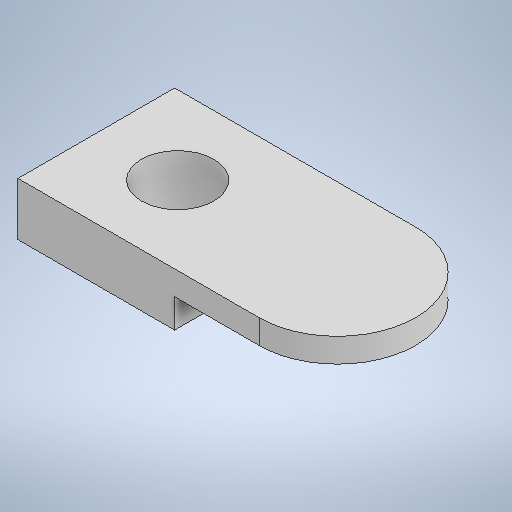
# Autodesk Inventor part: pinub
Saved by Autodesk Inventor 2025 (Build 290162000, 162)
## iProperties
Created: 2025-05-31
Part Number: pinub
Material: Generic
Document SubType Name: Modeling
Designer: ethan
Density: 1 g/cm^3
Appearance: Default
Author: ethan
Autodesk Inventor part; units mm, degrees
ref_plane "YZ Plane" through (0, 0, 0) normal (1, 0, 0) x (0, 1, 0)
ref_plane "XZ Plane" through (0, 0, 0) normal (0, 1, 0) x (-1, 0, 0)
ref_plane "XY Plane" through (0, 0, 0) normal (0, 0, 1) x (1, 0, 0)
sketch "Sketch1" plane through (0, 0, 0) normal (0, 1, 0) x (-1, 0, 0)
  line L0 (0, 0) -> (10, 0)
  line L1 (10, 0) -> (10, -6.5)
  line L2 (10, -6.5) -> (0, -6.5)
  line L3 (0, -6.5) -> (0, 0)
  arc A0 (0, 0) -> (0, -6.5) centre (0, -3.25) ccw
  dimension "d1" = 6.5
  dimension "d2" = 10
  constraints: 8 end point, 2 parallel, 2 point on circle, 2 tangent, 1 centre point, 1 horizontal, 1 perpendicular
  measures "d1" distance of L0.end L1.end
  measures "d2" distance of L1.end L2.end
extrude "Extrusion1" add sketch "Sketch1" along normal blind 1
sketch "Sketch2" plane through (0, 0, 0) normal (0, -1, 0) x (1, 0, 0)
  line L0 (-10, -6.5) -> (-10, 0) construction
  line L1 (0, -6.5) -> (-10, -6.5) construction
  arc A0 (0, -6.5) -> (0, 0) centre (0, -3.25) ccw construction
  line L2 (-10, 0) -> (0, 0) construction
  line L3 (-10, 0) -> (-3.5, 0) construction
  line L4 (-3.5, 0) -> (-3.5, -6.5) construction
  line L5 (-3.5, -6.5) -> (-10, -6.5) construction
  line L6 (-10, -6.5) -> (-10, 0) construction
  line L7 (-10, -3.25) -> (-6.625, -3.25) construction
  circle A1 centre (-6.625, -3.25) radius 1.5
  dimension "d5" = 6.5
  dimension "d6" = 3.375
  dimension "d7" = 3
  constraints: 10 end point, 2 horizontal, 2 parallel, 1 centre point, 1 coincident, 1 midpoint, 1 perpendicular, 1 point on line
  measures "d5" distance of L4.end L5.end
  measures "d6" distance of L7.start L7.end
  measures "d7" diameter of A1
extrude "Extrusion2" cut sketch "Sketch2" against normal blind 1
sketch "Sketch3" plane through (0, 0, 0) normal (0, -1, 0) x (1, 0, 0)
  circle A0 centre (-6.625, -3.25) radius 1.5 construction
  line L0 (-10, -6.5) -> (-10, 0) construction
  line L1 (0, -6.5) -> (-10, -6.5) construction
  arc A1 (0, -6.5) -> (0, 0) centre (0, -3.25) ccw construction
  line L2 (-10, 0) -> (0, 0) construction
  circle A2 centre (0, -3.25) radius 3.25 construction
  line L3 (-10, -6.5) -> (-3.5, -6.5)
  line L4 (-3.5, -6.5) -> (-3.5, 0)
  line L5 (-3.5, 0) -> (-10, 0)
  line L6 (-10, 0) -> (-10, -6.5)
  circle A3 centre (-6.625, -3.25) radius 1.5
  dimension "d10" = 6.5
  constraints: 8 end point, 2 coincident, 2 parallel, 1 centre point, 1 concentric, 1 horizontal, 1 perpendicular, 1 point on line, 1 vertical alignment, 2 other
  measures "d10" distance of L5.end L4.end
extrude "Extrusion3" add sketch "Sketch3" along normal blind 1.2
body "Solid1"
